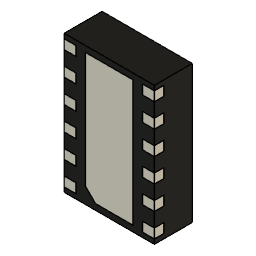
LM27762 (Autodesk Fusion 360 design; units mm, degrees)
Autodesk Fusion 360 part; units mm, degrees
sketch "草图1" plane through (0, 0, 0) normal (0, 1, 0) x (1, 0, 0)
  line L0 (-0.95, 1.45) -> (0.95, 1.45)
  line L1 (0.95, 1.45) -> (0.95, -1.45)
  line L2 (0.95, -1.45) -> (-0.95, -1.45)
  line L3 (-0.95, -1.45) -> (-0.95, 1.45)
  line L4 (-0.95, 1.45) -> (0.95, -1.45) construction
  line L5 (0.95, 1.45) -> (-0.95, -1.45) construction
  dimension "d1" = 2.9
  dimension "d2" = 1.9
  constraint horizontal L0
  constraint perpendicular L0 L1
  constraint parallel L0 L2
  constraint parallel L1 L3
  constraint coincident L4 origin
  constraint coincident L5 origin
  measures "d1" distance of L0.end L1.end
  measures "d2" distance of L1.end L2.end
extrude "拉伸1" add sketch "草图1" along normal blind 0.8 makes body 1
sketch "草图2" plane through (0, 0, 0) normal (0, -1, 0) x (1, 0, 0)
  line L0 (0.95, 1.45) -> (-0.95, 1.45)
  line L1 (-0.95, 1.45) -> (-0.95, -1.45)
  line L2 (-0.95, -1.45) -> (0.95, -1.45)
  line L3 (0.95, -1.45) -> (0.95, 1.45)
  line L4 (0, 2.5) -> (0, -3) construction
  line L5 (-2.5, 0) -> (3, 0) construction
  line L6 (-0.5, 1.325) -> (0.5, 1.325)
  line L7 (0.5, 1.325) -> (0.5, -1.325)
  line L8 (0.5, -1.325) -> (-0.2879, -1.325)
  line L9 (-0.2879, -1.325) -> (-0.5, -1.1129)
  line L10 (-0.5, -1.1129) -> (-0.5, 1.325)
  line L11 (-0.95, 1.35) -> (-0.7, 1.35)
  line L12 (-0.7, 1.35) -> (-0.7, 1.15)
  line L13 (-0.7, 1.15) -> (-0.95, 1.15)
  line L14 (-0.95, 1.15) -> (-0.95, 1.35)
  line L15 (-0.7, -1.15) -> (-0.95, -1.15)
  line L16 (-0.7, -1.35) -> (-0.7, -1.15)
  line L17 (-0.95, -1.15) -> (-0.95, -1.35)
  line L18 (-0.95, -1.35) -> (-0.7, -1.35)
  line L19 (-0.7, 0.65) -> (-0.95, 0.65)
  line L20 (-0.7, 0.85) -> (-0.7, 0.65)
  line L21 (-0.95, 0.85) -> (-0.7, 0.85)
  line L22 (-0.95, 0.65) -> (-0.95, 0.85)
  line L23 (-0.7, 0.15) -> (-0.95, 0.15)
  line L24 (-0.7, 0.35) -> (-0.7, 0.15)
  line L25 (-0.95, 0.35) -> (-0.7, 0.35)
  line L26 (-0.95, 0.15) -> (-0.95, 0.35)
  line L27 (-0.7, -0.35) -> (-0.95, -0.35)
  line L28 (-0.7, -0.15) -> (-0.7, -0.35)
  line L29 (-0.95, -0.15) -> (-0.7, -0.15)
  line L30 (-0.95, -0.35) -> (-0.95, -0.15)
  line L31 (-0.7, -0.85) -> (-0.95, -0.85)
  line L32 (-0.7, -0.65) -> (-0.7, -0.85)
  line L33 (-0.95, -0.65) -> (-0.7, -0.65)
  line L34 (-0.95, -0.85) -> (-0.95, -0.65)
  line L35 (-0.7, -1.35) -> (-0.95, -1.35)
  line L36 (-0.7, -1.15) -> (-0.7, -1.35)
  line L37 (-0.95, -1.15) -> (-0.7, -1.15)
  line L38 (-0.95, -1.35) -> (-0.95, -1.15)
  line L39 (0.7, 1.15) -> (0.95, 1.15)
  line L40 (0.7, 1.35) -> (0.7, 1.15)
  line L41 (0.95, 1.35) -> (0.7, 1.35)
  line L42 (0.95, 1.15) -> (0.95, 1.35)
  line L43 (0.95, 0.85) -> (0.7, 0.85)
  line L44 (0.7, 0.85) -> (0.7, 0.65)
  line L45 (0.7, 0.65) -> (0.95, 0.65)
  line L46 (0.95, 0.65) -> (0.95, 0.85)
  line L47 (0.95, 0.35) -> (0.7, 0.35)
  line L48 (0.7, 0.35) -> (0.7, 0.15)
  line L49 (0.7, 0.15) -> (0.95, 0.15)
  line L50 (0.95, 0.15) -> (0.95, 0.35)
  line L51 (0.95, -0.15) -> (0.7, -0.15)
  line L52 (0.7, -0.15) -> (0.7, -0.35)
  line L53 (0.7, -0.35) -> (0.95, -0.35)
  line L54 (0.95, -0.35) -> (0.95, -0.15)
  line L55 (0.95, -0.65) -> (0.7, -0.65)
  line L56 (0.7, -0.65) -> (0.7, -0.85)
  line L57 (0.7, -0.85) -> (0.95, -0.85)
  line L58 (0.95, -0.85) -> (0.95, -0.65)
  line L59 (0.7, -1.15) -> (0.95, -1.15)
  line L60 (0.7, -1.15) -> (0.7, -1.35)
  line L61 (0.95, -1.35) -> (0.95, -1.15)
  line L62 (0.95, -1.35) -> (0.7, -1.35)
  dimension "d5" = 1
  dimension "d6" = 2.65
  dimension "d7" = 135
  dimension "d8" = 0.3
  dimension "d9" = 0.2
  dimension "d10" = 0.25
  dimension "d11" = 2.7
  dimension "d14" = 0
  dimension "d15" = -2.5
  constraint vertical L4
  constraint perpendicular L1 L5
  constraint perpendicular L4 L6
  constraint perpendicular L6 L7
  constraint perpendicular L4 L8
  constraint perpendicular L6 L10
  constraint horizontal L11
  constraint vertical L12
  constraint horizontal L13
  constraint vertical L14
  constraint collinear L1 L14
  constraint symmetric L5 L11.start L17.end
  constraint symmetric L5 L11.end L16.start
  constraint symmetric L5 L12.end L15.start
  constraint symmetric L5 L13.end L15.end
  constraint symmetric L4 L11.start L41.start
  constraint symmetric L4 L11.end L40.start
  constraint symmetric L4 L12.end L39.start
  constraint symmetric L4 L13.end L39.end
  constraint symmetric L4 L15.start L59.start
  constraint symmetric L4 L15.end L59.end
  constraint symmetric L4 L16.start L60.end
  constraint symmetric L4 L17.end L61.start
  constraint symmetric L4 L19.start L44.end
  constraint symmetric L4 L19.end L45.end
  constraint symmetric L4 L20.start L43.end
  constraint symmetric L4 L21.start L43.start
  constraint symmetric L4 L23.start L48.end
  constraint symmetric L4 L23.end L49.end
  constraint symmetric L4 L24.start L47.end
  constraint symmetric L4 L25.start L47.start
  constraint symmetric L4 L27.start L52.end
  constraint symmetric L4 L27.end L53.end
  constraint symmetric L4 L28.start L51.end
  constraint symmetric L4 L29.start L51.start
  constraint symmetric L4 L31.start L56.end
  constraint symmetric L4 L31.end L57.end
  constraint symmetric L4 L32.start L55.end
  constraint symmetric L4 L33.start L55.start
  measures "d5" distance of L6.start L6.end
  measures "d6" distance of L6.end L7.end
  measures "d7" angle of L9 L10
  measures "d8" distance of L8.end L9.end
  measures "d9" distance of L11.start L13.end
  measures "d10" distance of L11.start L11.end
  measures "d11" distance of L11.start L17.end
extrude "拉伸2" cut sketch "草图2" against normal blind 0.2 contours L6 L7 L8 L9 L10 bodies 1
extrude "拉伸3" cut sketch "草图2" against normal blind 0.2 contours L3 L39 L40 L41 L42 | L1 L11 L12 L13 L14 | L3 L43 L44 L45 L46 | L1 L19 L20 L21 L22 | L3 L47 L48 L49 L50 | L1 L23 L24 L25 L26 | L3 L51 L52 L53 L54 | L1 L27 L28 L29 L30 | L3 L55 L56 L57 L58 | L1 L31 L32 L33 L34 | L3 L59 L60 L61 L62 | L1 L15 L16 L17 L18 L35 L36 L37 L38 bodies 1
extrude "拉伸4" add sketch "草图2" against normal blind 0.2 separate body contours L3 L39 L40 L41 L42 | L1 L11 L12 L13 L14 | L3 L43 L44 L45 L46 | L1 L19 L20 L21 L22 | L3 L47 L48 L49 L50 | L1 L23 L24 L25 L26 | L3 L51 L52 L53 L54 | L1 L27 L28 L29 L30 | L3 L55 L56 L57 L58 | L1 L31 L32 L33 L34 | L3 L59 L60 L61 L62 | L1 L15 L16 L17 L18 L35 L36 L37 L38 | L6 L7 L8 L9 L10 makes body 2 at (0.8667, 0, -0.7833) makes body 3 at (-0.8667, 0, -0.2167) makes body 4 at (-0.8667, 0, 0.7833) makes body 5 at (0.1667, 0, -0.371) makes body 6 at (-0.8667, 0, 0.2833) makes body 7 at (0.7833, 0, -1.2167) makes body 8 at (0.7833, 0, -0.2167) makes body 9 at (-0.8667, 0, -0.7167) makes body 10 at (0.8667, 0, 1.2167) makes body 11 at (-0.8667, 0, 1.2833) makes body 12 at (0.8667, 0, 0.7167) makes body 13 at (-0.8667, 0.0667, -1.35) makes body 14 at (0.8667, 0, 0.2167)
